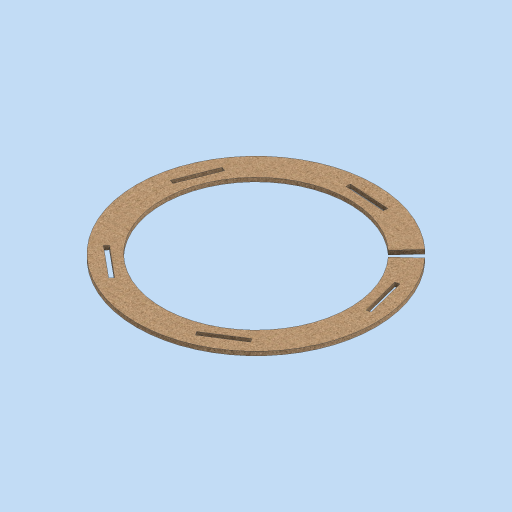
# Autodesk Inventor part: D14_CM_CIRCULO
Saved by Autodesk Inventor 2024.2 (Build 282272000, 272)
## iProperties
Created: 2024-10-01
Part Number: D14_CM_CIRCULO
Material: MDF Medium Density Fiberboard
Document SubType Name: Modeling
Designer: jrcer
Density: 0.8 g/cm^3
Appearance: Cardboard - Corrugated
Author: jrcer
Autodesk Inventor part; units mm, degrees
ref_plane "YZ Plane" through (0, 0, 0) normal (1, 0, 0) x (0, 1, 0)
ref_plane "XZ Plane" through (0, 0, 0) normal (0, 1, 0) x (-1, 0, 0)
ref_plane "XY Plane" through (0, 0, 0) normal (0, 0, 1) x (1, 0, 0)
sketch "Sketch1" plane through (0, 0, 0) normal (0, 1, 0) x (-1, 0, 0)
  circle A0 centre (0, 0) radius 70.5
  circle A1 centre (0, 0) radius 90
  line L0 (90, 0) -> (70.5, 0)
  line L1 (-90, 0) -> (-70.5, 0)
  line L2 (0, 0) -> (-70.5, 0) construction
  line L3 (0, 70.5) -> (0, 0) construction
  line L4 (0, 90) -> (0, 70.5)
  line L5 (-70.5, 0) -> (-90, 0)
  line L6 (-74.25, 7) -> (-86.25, 7)
  line L7 (-86.25, 7) -> (-83.7022, 0)
  line L8 (-74.25, 7) -> (-76.7978, 0)
  line L9 (-80.25, 0) -> (-80.25, 7) construction
  line L10 (-55.5838, 59.7031) -> (-30.242, 75.7591)
  line L11 (-30.242, 75.7591) -> (-28.5294, 73.056)
  line L12 (-28.5294, 73.056) -> (-53.8711, 57)
  line L13 (-53.8711, 57) -> (-55.5838, 59.7031)
  line L14 (-55.5838, 59.7031) -> (-28.5294, 73.056) construction
  line L15 (-30.242, 75.7591) -> (-53.8711, 57) construction
  circle A2 centre (0, 0) radius 80 construction
  line L16 (-73.9574, -34.414) -> (-81.3965, -5.351)
  line L17 (-70.8573, -33.6205) -> (-73.9574, -34.414)
  line L18 (-78.2964, -4.5575) -> (-70.8573, -33.6205)
  line L19 (-81.3965, -5.351) -> (-78.2964, -4.5575)
  line L20 (9.8756, -80.9722) -> (-20.0638, -79.0662)
  line L21 (10.0789, -77.7786) -> (9.8756, -80.9722)
  line L22 (-19.8605, -75.8727) -> (10.0789, -77.7786)
  line L23 (-20.0638, -79.0662) -> (-19.8605, -75.8727)
  line L24 (80.0608, -15.6295) -> (68.9964, -43.5146)
  line L25 (77.0864, -14.4493) -> (80.0608, -15.6295)
  line L26 (66.022, -42.3344) -> (77.0864, -14.4493)
  line L27 (68.9964, -43.5146) -> (66.022, -42.3344)
  line L28 (0, 0) -> (-63.6396, -63.6396) construction
  line L29 (0, 0) -> (-60.8031, -66.355)
  line L30 (0, 0) -> (-66.355, -60.8031)
  line L31 (39.6047, 71.3126) -> (62.7059, 52.1727)
  line L32 (37.5631, 68.8485) -> (39.6047, 71.3126)
  line L33 (60.6643, 49.7086) -> (37.5631, 68.8485)
  line L34 (62.7059, 52.1727) -> (60.6643, 49.7086)
  point P0 (80.25, 0)
  point P1 (-80.25, 0)
  point P2 (-42.0566, 66.3795)
  point P3 (-15.2947, 78.5243)
  point P4 (-54.7275, 58.3516)
  point P5 (-29.3857, 74.4075)
  point P6 (-72.4073, -34.0173)
  point P7 (-79.8464, -4.9543)
  point P8 (9.9773, -79.3754)
  point P9 (-19.9621, -77.4694)
  point P10 (78.5736, -15.0394)
  point P11 (67.5092, -42.9245)
  point P12 (-76.7978, 0)
  point P13 (-83.7022, 0)
  point P14 (38.5839, 70.0805)
  point P15 (61.6851, 50.9406)
  point P16 (-51.9781, -47.6291)
  point P17 (-47.6291, -51.9781)
  dimension "d1" = 180
  dimension "d0" = 141
  dimension "d4" = 90
  dimension "d5" = 7
  dimension "d6" = 70
  dimension "d8" = 12
  dimension "d13" = 3.2
  dimension "d14" = 30
  dimension "d15" = 50
  dimension "d20" = 160
  dimension "d27" = 360
  dimension "d29" = 45
  dimension "d32" = 5
  dimension "d33" = 2.5
  constraints: 70 end point, 8 midpoint, 7 point on circle, 3 coincident, 3 parallel, 2 centre point, 2 horizontal, 2 horizontal alignment, 2 perpendicular, 2 point on line, 2 vertical, 1 collinear, 1 equal length, 60 other
  measures "d0" diameter of A0
  measures "d4" angle of L2 L3
  measures "d5" distance between parallel lines of L6 L5
  measures "d6" angle of L7 L6
  measures "d8" distance of L6.start L6.end
  measures "d13" distance of L10.end L11.end
  measures "d14" distance of L11.end L12.end
  measures "d15" vertical distance of L12.end L6.start
  measures "d20" diameter of A2
  measures "d29" angle of L5 L28
  measures "d32" angle of L30 L29
  measures "d33" angle of L30 L28
extrude "Extrusion1" add sketch "Sketch1" along normal blind 3 contours L0 A1 L29 A0 | A0 L4 A1 L0 | A0 L1 L8 L6 L7 A1 L4 | A0 L30 A1 L1 | L1 L7 L6 L8
equation "\"d33\" = 0.5 * d32"
body "Solid1"
